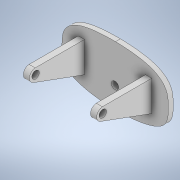
# Autodesk Inventor part: head_mount
Saved by Autodesk Inventor 2020.3 (Build 243373000, 373)
## iProperties
Created: 2020-08-24
Part Number: head_mount
Material: Generic
Document SubType Name: Modeling
Designer: aditk
Density: 1 g/cm^3
Appearance: Default
Author: aditk
Autodesk Inventor part; units mm, degrees
ref_plane "YZ Plane" through (0, 0, 0) normal (1, 0, 0) x (0, 1, 0)
ref_plane "XZ Plane" through (0, 0, 0) normal (0, 1, 0) x (-1, 0, 0)
ref_plane "XY Plane" through (0, 0, 0) normal (0, 0, 1) x (1, 0, 0)
sketch "Sketch1" plane through (0, 0, 0) normal (0, 0, 1) x (1, 0, 0)
  spline S0 degree 3 poles (-0.2094, -17.1721) (6.9132, -17.2293) (16.1793, -16.6609) (25.7819, -14.763) (30.1768, -13.5581) (34.0622, -12.0843) (37.3356, -10.329) (39.8919, -8.2788) (41.6355, -5.9236) (42.7249, -3.3486) (43.3094, -0.6356) (43.5427, 2.1317) (43.5699, 4.8733) (43.5663, 7.4972) (43.4971, 10.8173) (43.153, 13.8943) (42.2346, 16.7548) (41.1833, 18.7987) (39.7719, 20.7225) (37.4099, 23.1038) (33.5585, 25.6882) (27.5013, 28.0303) (19.9992, 29.6922) (11.0435, 30.7417) (4.0981, 31.0803) (0.3802, 31.171) knots 0 0 0 0 0.125 0.15625 0.1875 0.21875 0.25 0.28125 0.3125 0.34375 0.375 0.40625 0.4375 0.46875 0.5 0.5625 0.59375 0.625 0.65625 0.6875 0.75 0.8125 0.875 0.9375 1 1 1 1
  circle A0 centre (0, 0) radius 3
  spline S1 degree 3 poles (-0.2094, -17.1721) (-7.3314, -17.0556) (-16.5809, -16.2614) (-26.1343, -14.1299) (-30.4985, -12.8181) (-34.3468, -11.25) (-37.5764, -9.4154) (-40.0819, -7.3035) (-41.7676, -4.9064) (-42.7939, -2.3056) (-43.312, 0.4208) (-43.4777, 3.193) (-43.4382, 5.9344) (-43.3706, 8.5574) (-43.2204, 11.8749) (-42.8014, 14.9426) (-41.8134, 17.7798) (-40.7126, 19.7975) (-39.2547, 21.6863) (-36.8353, 24.0093) (-32.9221, 26.499) (-26.8095, 28.6926) (-19.2692, 30.1711) (-10.2905, 31.0019) (-3.3389, 31.171) (0.3802, 31.171) knots 0 0 0 0 0.125 0.15625 0.1875 0.21875 0.25 0.28125 0.3125 0.34375 0.375 0.40625 0.4375 0.46875 0.5 0.5625 0.59375 0.625 0.65625 0.6875 0.75 0.8125 0.875 0.9375 1 1 1 1
  point P0 (30.4031, 301.1702)
  constraints: 1 centre point, 4 other
extrude "Extrusion1" add sketch "Sketch1" along normal blind 4
sketch "Sketch2" plane through (0, 0, 4) normal (0, 0, 1) x (1, 0, 0)
  line L0 (0, 0) -> (-30, 0)
  line L1 (-30, 0) -> (-30, 10)
  line L2 (-30, 10) -> (-30, 20)
  line L3 (-30, 20) -> (30, 20)
  line L4 (30, 20) -> (30, 0)
  line L5 (30, 0) -> (30, -5)
  line L6 (30, -5) -> (-30, -5)
  line L7 (-30, -5) -> (-30, 0)
  line L8 (-30, -5) -> (-25, -5)
  line L9 (-25, -5) -> (-25, 20)
  line L10 (30, -5) -> (25, -5)
  line L11 (25, -5) -> (25, 20)
  line L12 (-30, 20) -> (-25, 20)
  line L13 (-25, 20) -> (-25, -5)
  line L14 (-25, -5) -> (-30, -5)
  line L15 (-30, -5) -> (-30, 20)
  line L16 (25, 20) -> (30, 20)
  line L17 (30, 20) -> (30, -5)
  line L18 (30, -5) -> (25, -5)
  line L19 (25, -5) -> (25, 20)
  constraints: 40 end point, 8 perpendicular, 6 point on line, 4 horizontal, 4 parallel
extrude "Extrusion2" add sketch "Sketch2" along normal blind 50 contours L9 L6 L7 L0 | L0 L1 L2 L3 L9 | L11 L3 L4 L5 L6
sketch "Sketch3" plane through (30, -5, 4) normal (1, 0, 0) x (0, 0, -1)
  line L0 (0, 0) -> (-40, 0)
  line L1 (-40, 0) -> (-40, 20)
  line L2 (-40, 20) -> (0, 20)
  line L3 (0, 20) -> (0, 0)
  circle A0 centre (-40, 20) radius 5.0104
  line L4 (0, 0) -> (-50, 0) projected
  line L5 (0, 0) -> (-41.7245, 15.2957)
  circle A1 centre (-40, 20) radius 3
  line L6 (0, 25) -> (0, 0) projected
  line L7 (0, 25) -> (-50, 25) projected
  line L8 (-50, 0) -> (-50, 25) projected
  line L9 (0, 0) -> (-50, 0) projected
  line L10 (0, 25) -> (-50, 25) projected
  line L11 (-50, 25) -> (4, 25)
  line L12 (4, 25) -> (4, 0)
  line L13 (4, 0) -> (-50, 0)
  line L14 (-50, 0) -> (-50, 25)
  point P0 (4, 5)
  point P1 (-40.3226, 25)
  dimension "d11" = 40
  dimension "d12" = 20
  dimension "d13" = 6
  constraints: 18 end point, 4 parallel, 2 coincident, 2 horizontal, 2 perpendicular, 1 centre point, 4 other
  measures "d11" distance of L1.end L2.end
  measures "d12" distance of L0.end L1.end
  measures "d13" diameter of A1
extrude "Extrusion3" cut sketch "Sketch3" against normal through all contours L0 L1 L5 | L4 L8 L7 A0 L5 L1 | A1 L1 L2 | L2 L1 A1
body "Solid1"
